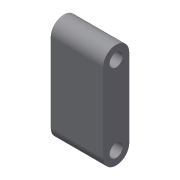
# Autodesk Inventor part: Tank Tread link B
Saved by Autodesk Inventor 2015 (Build 190159000, 159)
## iProperties
Created: 2015-03-14
Part Number: Tank Tread link B
Material: Generic
Document SubType Name: Modeling
Designer: james_000
Density: 1 g/cm^3
Appearance: Default
Author: james_000
Autodesk Inventor part; units mm, degrees
ref_plane "YZ Plane" through (0, 0, 0) normal (1, 0, 0) x (0, 1, 0)
ref_plane "XZ Plane" through (0, 0, 0) normal (0, 1, 0) x (-1, 0, 0)
ref_plane "XY Plane" through (0, 0, 0) normal (0, 0, 1) x (1, 0, 0)
sketch "Sketch2" plane through (0, 0, 0) normal (1, 0, 0) x (0, 1, 0)
  arc A0 (0.5, 0) -> (-0.5, 0) centre (0, 0) ccw
  circle A1 centre (0, 0) radius 0.25
  circle A2 centre (0, -3) radius 0.25
  arc A3 (-0.5, -3) -> (0.5, -3) centre (0, -3) ccw
  line L0 (0.5, 0) -> (0.5, -3)
  line L1 (-0.5, 0) -> (-0.5, -3)
  dimension "d7" = 1
  dimension "d8" = 0.5
  dimension "d10" = 0.5
  dimension "d11" = 1
  constraints: 4 centre point, 4 end point, 4 point on circle, 3 coincident, 2 tangent
  measures "d7" diameter of A0
  measures "d8" diameter of A1
  measures "d10" diameter of A2
  measures "d11" diameter of A3
extrude "Extrusion2" add sketch "Sketch2" along normal blind 2
body "Solid2"
